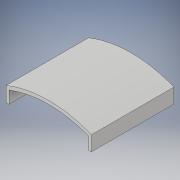
# Autodesk Inventor part: Canopy
Saved by Autodesk Inventor 2019 (Build 230136000, 136)
## iProperties
Created: 2019-01-12
Part Number: Canopy
Material: Generic
Document SubType Name: Modeling
Designer: User
Density: 1 g/cm^3
Appearance: Default
Author: User
Autodesk Inventor part; units mm, degrees
ref_plane "YZ Plane" through (0, 0, 0) normal (1, 0, 0) x (0, 1, 0)
ref_plane "XZ Plane" through (0, 0, 0) normal (0, 1, 0) x (-1, 0, 0)
ref_plane "XY Plane" through (0, 0, 0) normal (0, 0, 1) x (1, 0, 0)
sketch "Sketch1" plane through (0, 0, 0) normal (0, 0, 1) x (1, 0, 0)
  line L0 (0, 0) -> (3.175, 0)
  line L1 (3.175, 0) -> (3.175, 12.7)
  line L2 (3.175, 12.7) -> (0, 12.7)
  line L3 (0, 12.7) -> (0, 0)
  line L4 (84.963, 0) -> (88.138, 0)
  line L5 (88.138, 0) -> (88.138, 12.7)
  line L6 (88.138, 12.7) -> (84.963, 12.7)
  line L7 (84.963, 12.7) -> (84.963, 0)
  arc A0 (84.963, 12.7) -> (3.175, 12.7) centre (44.069, -94.3642) ccw
  line L8 (0, 12.7) -> (0, 15.2331)
  line L9 (88.138, 12.7) -> (88.138, 15.2331)
  arc A1 (88.138, 15.2331) -> (0, 15.2331) centre (44.069, -94.3642) ccw
  dimension "d0" = 3.175
  dimension "d1" = 12.7
  dimension "d2" = 81.788
  dimension "d3" = 3.175
  dimension "d4" = 12.7
  dimension "d5" = 2.5331
  dimension "d6" = 2.5331
  constraints: 20 end point, 4 parallel, 4 point on circle, 2 centre point, 2 horizontal, 2 perpendicular, 2 vertical, 1 concentric
  measures "d0" distance of L2.end L1.end
  measures "d1" distance of L1.end L0.end
  measures "d2" distance of L4.start L0.end
  measures "d3" distance between parallel lines of L5 L7
  measures "d4" distance of L4.end L5.end
  measures "d5" distance of L5.end L9.end
  measures "d6" distance of L2.end L8.end
extrude "Extrusion1" add sketch "Sketch1" along normal blind 85.09
equation "\"d3\" = d0"
equation "\"d4\" = d1"
equation "\"d6\" = d5"
body "Solid1"
